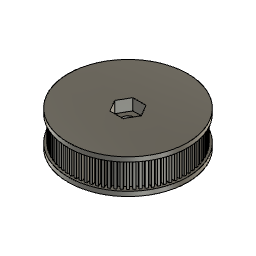
pulley5080 (Autodesk Fusion 360 design; units mm, degrees)
Autodesk Fusion 360 part; units mm, degrees
sketch "Sketch1" plane through (0, 0, 0) normal (0, 0, 1) x (1, 0, 0)
  line L0 (0.5, 23.5) -> (0.5, 25)
  line L1 (0.5, 25) -> (-0.5, 25)
  line L2 (-0.5, 25) -> (-0.5, 23.5)
  line L3 (0, 1.75) -> (0, 22.5)
  circle A0 centre (0, 0) radius 23.5053
  line L4 (-2.4599, 24.8837) -> (-2.3422, 23.3883)
  line L5 (-1.463, 24.9622) -> (-2.4599, 24.8837)
  line L6 (-1.3453, 23.4668) -> (-1.463, 24.9622)
  line L7 (-4.4047, 24.614) -> (-4.1701, 23.1325)
  line L8 (-3.417, 24.7704) -> (-4.4047, 24.614)
  line L9 (-3.1824, 23.2889) -> (-3.417, 24.7704)
  line L10 (-6.3223, 24.1925) -> (-5.9722, 22.734)
  line L11 (-5.3499, 24.426) -> (-6.3223, 24.1925)
  line L12 (-4.9998, 22.9674) -> (-5.3499, 24.426)
  line L13 (-8.201, 23.6219) -> (-7.7374, 22.1953)
  line L14 (-7.2499, 23.9309) -> (-8.201, 23.6219)
  line L15 (-6.7864, 22.5043) -> (-7.2499, 23.9309)
  line L16 (-10.029, 22.9056) -> (-9.455, 21.5198)
  line L17 (-9.1051, 23.2883) -> (-10.029, 22.9056)
  line L18 (-8.5311, 21.9025) -> (-9.1051, 23.2883)
  line L19 (-11.7953, 22.0482) -> (-11.1143, 20.7117)
  line L20 (-10.9043, 22.5022) -> (-11.7953, 22.0482)
  line L21 (-10.2233, 21.1656) -> (-10.9043, 22.5022)
  line L22 (-13.4888, 21.0548) -> (-12.705, 19.7758)
  line L23 (-12.6361, 21.5773) -> (-13.4888, 21.0548)
  line L24 (-11.8524, 20.2983) -> (-12.6361, 21.5773)
  line L25 (-15.0991, 19.9315) -> (-14.2175, 18.718)
  line L26 (-14.2901, 20.5193) -> (-15.0991, 19.9315)
  line L27 (-13.4084, 19.3058) -> (-14.2901, 20.5193)
  line L28 (-16.6164, 18.6854) -> (-15.6422, 17.5448)
  line L29 (-15.856, 19.3349) -> (-16.6164, 18.6854)
  line L30 (-14.8818, 18.1943) -> (-15.856, 19.3349)
  line L31 (-18.0312, 17.3241) -> (-16.9706, 16.2635)
  line L32 (-17.3241, 18.0312) -> (-18.0312, 17.3241)
  line L33 (-16.2635, 16.9706) -> (-17.3241, 18.0312)
  line L34 (-19.3349, 15.856) -> (-18.1943, 14.8818)
  line L35 (-18.6854, 16.6164) -> (-19.3349, 15.856)
  line L36 (-17.5448, 15.6422) -> (-18.6854, 16.6164)
  line L37 (-20.5193, 14.2901) -> (-19.3058, 13.4084)
  line L38 (-19.9315, 15.0991) -> (-20.5193, 14.2901)
  line L39 (-18.718, 14.2175) -> (-19.9315, 15.0991)
  line L40 (-21.5773, 12.6361) -> (-20.2983, 11.8524)
  line L41 (-21.0548, 13.4888) -> (-21.5773, 12.6361)
  line L42 (-19.7758, 12.705) -> (-21.0548, 13.4888)
  line L43 (-22.5022, 10.9043) -> (-21.1656, 10.2233)
  line L44 (-22.0482, 11.7953) -> (-22.5022, 10.9043)
  line L45 (-20.7117, 11.1143) -> (-22.0482, 11.7953)
  line L46 (-23.2883, 9.1051) -> (-21.9025, 8.5311)
  line L47 (-22.9056, 10.029) -> (-23.2883, 9.1051)
  line L48 (-21.5198, 9.455) -> (-22.9056, 10.029)
  line L49 (-23.9309, 7.2499) -> (-22.5043, 6.7864)
  line L50 (-23.6219, 8.201) -> (-23.9309, 7.2499)
  line L51 (-22.1953, 7.7374) -> (-23.6219, 8.201)
  line L52 (-24.426, 5.3499) -> (-22.9674, 4.9998)
  line L53 (-24.1925, 6.3223) -> (-24.426, 5.3499)
  line L54 (-22.734, 5.9722) -> (-24.1925, 6.3223)
  line L55 (-24.7704, 3.417) -> (-23.2889, 3.1824)
  line L56 (-24.614, 4.4047) -> (-24.7704, 3.417)
  line L57 (-23.1325, 4.1701) -> (-24.614, 4.4047)
  line L58 (-24.9622, 1.463) -> (-23.4668, 1.3453)
  line L59 (-24.8837, 2.4599) -> (-24.9622, 1.463)
  line L60 (-23.3883, 2.3422) -> (-24.8837, 2.4599)
  line L61 (-25, -0.5) -> (-23.5, -0.5)
  line L62 (-25, 0.5) -> (-25, -0.5)
  line L63 (-23.5, 0.5) -> (-25, 0.5)
  line L64 (-24.8837, -2.4599) -> (-23.3883, -2.3422)
  line L65 (-24.9622, -1.463) -> (-24.8837, -2.4599)
  line L66 (-23.4668, -1.3453) -> (-24.9622, -1.463)
  line L67 (-24.614, -4.4047) -> (-23.1325, -4.1701)
  line L68 (-24.7704, -3.417) -> (-24.614, -4.4047)
  line L69 (-23.2889, -3.1824) -> (-24.7704, -3.417)
  line L70 (-24.1925, -6.3223) -> (-22.734, -5.9722)
  line L71 (-24.426, -5.3499) -> (-24.1925, -6.3223)
  line L72 (-22.9674, -4.9998) -> (-24.426, -5.3499)
  line L73 (-23.6219, -8.201) -> (-22.1953, -7.7374)
  line L74 (-23.9309, -7.2499) -> (-23.6219, -8.201)
  line L75 (-22.5043, -6.7864) -> (-23.9309, -7.2499)
  line L76 (-22.9056, -10.029) -> (-21.5198, -9.455)
  line L77 (-23.2883, -9.1051) -> (-22.9056, -10.029)
  line L78 (-21.9025, -8.5311) -> (-23.2883, -9.1051)
  line L79 (-22.0482, -11.7953) -> (-20.7117, -11.1143)
  line L80 (-22.5022, -10.9043) -> (-22.0482, -11.7953)
  line L81 (-21.1656, -10.2233) -> (-22.5022, -10.9043)
  line L82 (-21.0548, -13.4888) -> (-19.7758, -12.705)
  line L83 (-21.5773, -12.6361) -> (-21.0548, -13.4888)
  line L84 (-20.2983, -11.8524) -> (-21.5773, -12.6361)
  line L85 (-19.9315, -15.0991) -> (-18.718, -14.2175)
  line L86 (-20.5193, -14.2901) -> (-19.9315, -15.0991)
  line L87 (-19.3058, -13.4084) -> (-20.5193, -14.2901)
  line L88 (-18.6854, -16.6164) -> (-17.5448, -15.6422)
  line L89 (-19.3349, -15.856) -> (-18.6854, -16.6164)
  line L90 (-18.1943, -14.8818) -> (-19.3349, -15.856)
  line L91 (-17.3241, -18.0312) -> (-16.2635, -16.9706)
  line L92 (-18.0312, -17.3241) -> (-17.3241, -18.0312)
  line L93 (-16.9706, -16.2635) -> (-18.0312, -17.3241)
  line L94 (-15.856, -19.3349) -> (-14.8818, -18.1943)
  line L95 (-16.6164, -18.6854) -> (-15.856, -19.3349)
  line L96 (-15.6422, -17.5448) -> (-16.6164, -18.6854)
  line L97 (-14.2901, -20.5193) -> (-13.4084, -19.3058)
  line L98 (-15.0991, -19.9315) -> (-14.2901, -20.5193)
  line L99 (-14.2175, -18.718) -> (-15.0991, -19.9315)
  line L100 (-12.6361, -21.5773) -> (-11.8524, -20.2983)
  line L101 (-13.4888, -21.0548) -> (-12.6361, -21.5773)
  line L102 (-12.705, -19.7758) -> (-13.4888, -21.0548)
  line L103 (-10.9043, -22.5022) -> (-10.2233, -21.1656)
  line L104 (-11.7953, -22.0482) -> (-10.9043, -22.5022)
  line L105 (-11.1143, -20.7117) -> (-11.7953, -22.0482)
  line L106 (-9.1051, -23.2883) -> (-8.5311, -21.9025)
  line L107 (-10.029, -22.9056) -> (-9.1051, -23.2883)
  line L108 (-9.455, -21.5198) -> (-10.029, -22.9056)
  line L109 (-7.2499, -23.9309) -> (-6.7864, -22.5043)
  line L110 (-8.201, -23.6219) -> (-7.2499, -23.9309)
  line L111 (-7.7374, -22.1953) -> (-8.201, -23.6219)
  line L112 (-5.3499, -24.426) -> (-4.9998, -22.9674)
  line L113 (-6.3223, -24.1925) -> (-5.3499, -24.426)
  line L114 (-5.9722, -22.734) -> (-6.3223, -24.1925)
  line L115 (-3.417, -24.7704) -> (-3.1824, -23.2889)
  line L116 (-4.4047, -24.614) -> (-3.417, -24.7704)
  line L117 (-4.1701, -23.1325) -> (-4.4047, -24.614)
  line L118 (-1.463, -24.9622) -> (-1.3453, -23.4668)
  line L119 (-2.4599, -24.8837) -> (-1.463, -24.9622)
  line L120 (-2.3422, -23.3883) -> (-2.4599, -24.8837)
  line L121 (0.5, -25) -> (0.5, -23.5)
  line L122 (-0.5, -25) -> (0.5, -25)
  line L123 (-0.5, -23.5) -> (-0.5, -25)
  line L124 (2.4599, -24.8837) -> (2.3422, -23.3883)
  line L125 (1.463, -24.9622) -> (2.4599, -24.8837)
  line L126 (1.3453, -23.4668) -> (1.463, -24.9622)
  line L127 (4.4047, -24.614) -> (4.1701, -23.1325)
  line L128 (3.417, -24.7704) -> (4.4047, -24.614)
  line L129 (3.1824, -23.2889) -> (3.417, -24.7704)
  line L130 (6.3223, -24.1925) -> (5.9722, -22.734)
  line L131 (5.3499, -24.426) -> (6.3223, -24.1925)
  line L132 (4.9998, -22.9674) -> (5.3499, -24.426)
  line L133 (8.201, -23.6219) -> (7.7374, -22.1953)
  line L134 (7.2499, -23.9309) -> (8.201, -23.6219)
  line L135 (6.7864, -22.5043) -> (7.2499, -23.9309)
  line L136 (10.029, -22.9056) -> (9.455, -21.5198)
  line L137 (9.1051, -23.2883) -> (10.029, -22.9056)
  line L138 (8.5311, -21.9025) -> (9.1051, -23.2883)
  line L139 (11.7953, -22.0482) -> (11.1143, -20.7117)
  line L140 (10.9043, -22.5022) -> (11.7953, -22.0482)
  line L141 (10.2233, -21.1656) -> (10.9043, -22.5022)
  line L142 (13.4888, -21.0548) -> (12.705, -19.7758)
  line L143 (12.6361, -21.5773) -> (13.4888, -21.0548)
  line L144 (11.8524, -20.2983) -> (12.6361, -21.5773)
  line L145 (15.0991, -19.9315) -> (14.2175, -18.718)
  line L146 (14.2901, -20.5193) -> (15.0991, -19.9315)
  line L147 (13.4084, -19.3058) -> (14.2901, -20.5193)
  line L148 (16.6164, -18.6854) -> (15.6422, -17.5448)
  line L149 (15.856, -19.3349) -> (16.6164, -18.6854)
  line L150 (14.8818, -18.1943) -> (15.856, -19.3349)
  line L151 (18.0312, -17.3241) -> (16.9706, -16.2635)
  line L152 (17.3241, -18.0312) -> (18.0312, -17.3241)
  line L153 (16.2635, -16.9706) -> (17.3241, -18.0312)
  line L154 (19.3349, -15.856) -> (18.1943, -14.8818)
  line L155 (18.6854, -16.6164) -> (19.3349, -15.856)
  line L156 (17.5448, -15.6422) -> (18.6854, -16.6164)
  line L157 (20.5193, -14.2901) -> (19.3058, -13.4084)
  line L158 (19.9315, -15.0991) -> (20.5193, -14.2901)
  line L159 (18.718, -14.2175) -> (19.9315, -15.0991)
  line L160 (21.5773, -12.6361) -> (20.2983, -11.8524)
  line L161 (21.0548, -13.4888) -> (21.5773, -12.6361)
  line L162 (19.7758, -12.705) -> (21.0548, -13.4888)
  line L163 (22.5022, -10.9043) -> (21.1656, -10.2233)
  line L164 (22.0482, -11.7953) -> (22.5022, -10.9043)
  line L165 (20.7117, -11.1143) -> (22.0482, -11.7953)
  line L166 (23.2883, -9.1051) -> (21.9025, -8.5311)
  line L167 (22.9056, -10.029) -> (23.2883, -9.1051)
  line L168 (21.5198, -9.455) -> (22.9056, -10.029)
  line L169 (23.9309, -7.2499) -> (22.5043, -6.7864)
  line L170 (23.6219, -8.201) -> (23.9309, -7.2499)
  line L171 (22.1953, -7.7374) -> (23.6219, -8.201)
  line L172 (24.426, -5.3499) -> (22.9674, -4.9998)
  line L173 (24.1925, -6.3223) -> (24.426, -5.3499)
  line L174 (22.734, -5.9722) -> (24.1925, -6.3223)
  line L175 (24.7704, -3.417) -> (23.2889, -3.1824)
  line L176 (24.614, -4.4047) -> (24.7704, -3.417)
  line L177 (23.1325, -4.1701) -> (24.614, -4.4047)
  line L178 (24.9622, -1.463) -> (23.4668, -1.3453)
  line L179 (24.8837, -2.4599) -> (24.9622, -1.463)
  line L180 (23.3883, -2.3422) -> (24.8837, -2.4599)
  line L181 (25, 0.5) -> (23.5, 0.5)
  line L182 (25, -0.5) -> (25, 0.5)
  line L183 (23.5, -0.5) -> (25, -0.5)
  line L184 (24.8837, 2.4599) -> (23.3883, 2.3422)
  line L185 (24.9622, 1.463) -> (24.8837, 2.4599)
  line L186 (23.4668, 1.3453) -> (24.9622, 1.463)
  line L187 (24.614, 4.4047) -> (23.1325, 4.1701)
  line L188 (24.7704, 3.417) -> (24.614, 4.4047)
  line L189 (23.2889, 3.1824) -> (24.7704, 3.417)
  line L190 (24.1925, 6.3223) -> (22.734, 5.9722)
  line L191 (24.426, 5.3499) -> (24.1925, 6.3223)
  line L192 (22.9674, 4.9998) -> (24.426, 5.3499)
  line L193 (23.6219, 8.201) -> (22.1953, 7.7374)
  line L194 (23.9309, 7.2499) -> (23.6219, 8.201)
  line L195 (22.5043, 6.7864) -> (23.9309, 7.2499)
  line L196 (22.9056, 10.029) -> (21.5198, 9.455)
  line L197 (23.2883, 9.1051) -> (22.9056, 10.029)
  line L198 (21.9025, 8.5311) -> (23.2883, 9.1051)
  line L199 (22.0482, 11.7953) -> (20.7117, 11.1143)
  line L200 (22.5022, 10.9043) -> (22.0482, 11.7953)
  line L201 (21.1656, 10.2233) -> (22.5022, 10.9043)
  line L202 (21.0548, 13.4888) -> (19.7758, 12.705)
  line L203 (21.5773, 12.6361) -> (21.0548, 13.4888)
  line L204 (20.2983, 11.8524) -> (21.5773, 12.6361)
  line L205 (19.9315, 15.0991) -> (18.718, 14.2175)
  line L206 (20.5193, 14.2901) -> (19.9315, 15.0991)
  line L207 (19.3058, 13.4084) -> (20.5193, 14.2901)
  line L208 (18.6854, 16.6164) -> (17.5448, 15.6422)
  line L209 (19.3349, 15.856) -> (18.6854, 16.6164)
  line L210 (18.1943, 14.8818) -> (19.3349, 15.856)
  line L211 (17.3241, 18.0312) -> (16.2635, 16.9706)
  line L212 (18.0312, 17.3241) -> (17.3241, 18.0312)
  line L213 (16.9706, 16.2635) -> (18.0312, 17.3241)
  line L214 (15.856, 19.3349) -> (14.8818, 18.1943)
  line L215 (16.6164, 18.6854) -> (15.856, 19.3349)
  line L216 (15.6422, 17.5448) -> (16.6164, 18.6854)
  line L217 (14.2901, 20.5193) -> (13.4084, 19.3058)
  line L218 (15.0991, 19.9315) -> (14.2901, 20.5193)
  line L219 (14.2175, 18.718) -> (15.0991, 19.9315)
  line L220 (12.6361, 21.5773) -> (11.8524, 20.2983)
  line L221 (13.4888, 21.0548) -> (12.6361, 21.5773)
  line L222 (12.705, 19.7758) -> (13.4888, 21.0548)
  line L223 (10.9043, 22.5022) -> (10.2233, 21.1656)
  line L224 (11.7953, 22.0482) -> (10.9043, 22.5022)
  line L225 (11.1143, 20.7117) -> (11.7953, 22.0482)
  line L226 (9.1051, 23.2883) -> (8.5311, 21.9025)
  line L227 (10.029, 22.9056) -> (9.1051, 23.2883)
  line L228 (9.455, 21.5198) -> (10.029, 22.9056)
  line L229 (7.2499, 23.9309) -> (6.7864, 22.5043)
  line L230 (8.201, 23.6219) -> (7.2499, 23.9309)
  line L231 (7.7374, 22.1953) -> (8.201, 23.6219)
  line L232 (5.3499, 24.426) -> (4.9998, 22.9674)
  line L233 (6.3223, 24.1925) -> (5.3499, 24.426)
  line L234 (5.9722, 22.734) -> (6.3223, 24.1925)
  line L235 (3.417, 24.7704) -> (3.1824, 23.2889)
  line L236 (4.4047, 24.614) -> (3.417, 24.7704)
  line L237 (4.1701, 23.1325) -> (4.4047, 24.614)
  line L238 (1.463, 24.9622) -> (1.3453, 23.4668)
  line L239 (2.4599, 24.8837) -> (1.463, 24.9622)
  line L240 (2.3422, 23.3883) -> (2.4599, 24.8837)
  circle A1 centre (0, 0) radius 26
  dimension "d1" = 1
  dimension "d2" = 1.5
  dimension "d3" = 25
  dimension "d5" = 360
  dimension "d6" = 52
  constraint vertical L0
  constraint horizontal L1
  constraint vertical L2
  constraint symmetric L2.end L0.start L3
  constraint coincident A0.centre A1.centre
  constraint coincident L2.end A0
  measures "d1" distance of L0.end L1.end
  measures "d2" distance of L0.start L0.end
  measures "d3" distance of A0.centre L1
  measures "d6" diameter of A1
extrude "Extrude1" add sketch "Sketch1" along normal blind 15 contours L0 L1 L2 A0 | A0 | A0 L238 L239 L240 | A0 L4 L5 L6 | A0 L235 L236 L237 | A0 L7 L8 L9 | A0 L232 L233 L234 | A0 L10 L11 L12 | A0 L229 L230 L231 | A0 L13 L14 L15 | A0 L226 L227 L228 | A0 L16 L17 L18 | A0 L223 L224 L225 | A0 L19 L20 L21 | A0 L220 L221 L222 | A0 L22 L23 L24 | A0 L217 L218 L219 | A0 L25 L26 L27 | A0 L214 L215 L216 | A0 L28 L29 L30 | A0 L211 L212 L213 | A0 L31 L32 L33 | A0 L208 L209 L210 | A0 L34 L35 L36 | A0 L205 L206 L207 | A0 L37 L38 L39 | A0 L202 L203 L204 | A0 L40 L41 L42 | A0 L199 L200 L201 | A0 L43 L44 L45 | A0 L196 L197 L198 | A0 L46 L47 L48 | A0 L193 L194 L195 | A0 L49 L50 L51 | A0 L190 L191 L192 | A0 L52 L53 L54 | A0 L187 L188 L189 | A0 L55 L56 L57 | A0 L184 L185 L186 | A0 L58 L59 L60 | A0 L181 L182 L183 | A0 L61 L62 L63 | A0 L178 L179 L180 | A0 L64 L65 L66 | A0 L175 L176 L177 | A0 L67 L68 L69 | A0 L172 L173 L174 | A0 L70 L71 L72 | A0 L169 L170 L171 | A0 L73 L74 L75 | A0 L166 L167 L168 | A0 L76 L77 L78 | A0 L163 L164 L165 | A0 L79 L80 L81 | A0 L160 L161 L162 | A0 L82 L83 L84 | A0 L157 L158 L159 | A0 L85 L86 L87 | A0 L154 L155 L156 | A0 L88 L89 L90 | A0 L151 L152 L153 | A0 L91 L92 L93 | A0 L148 L149 L150 | A0 L94 L95 L96 | A0 L145 L146 L147 | A0 L97 L98 L99 | A0 L142 L143 L144 | A0 L100 L101 L102 | A0 L139 L140 L141 | A0 L103 L104 L105 | A0 L136 L137 L138 | A0 L106 L107 L108 | A0 L133 L134 L135 | A0 L109 L110 L111 | A0 L130 L131 L132 | A0 L112 L113 L114 | A0 L127 L128 L129 | A0 L115 L116 L117 | A0 L124 L125 L126 | A0 L118 L119 L120 | A0 L121 L122 L123
extrude "Extrude2" add sketch "Sketch1" along normal blind 2
extrude "Extrude3" add sketch "Sketch1" against normal blind 2 from surface at 15
sketch "Sketch2" plane through (0, 0, 15) normal (0, 0, 1) x (-1, 0, 0)
  circle A0 centre (0, 0) radius 26
  circle A1 centre (0, 0) radius 3
  line L0 (2.8868, -5) -> (5.7735, 0)
  line L1 (5.7735, 0) -> (2.8868, 5)
  line L2 (2.8868, 5) -> (-2.8868, 5)
  line L3 (-2.8868, 5) -> (-5.7735, 0)
  line L4 (-5.7735, 0) -> (-2.8868, -5)
  line L5 (-2.8868, -5) -> (2.8868, -5)
  dimension "d14" = 6
  dimension "d15" = 10
  constraint coincident A0.centre A1.centre
  constraint horizontal L5
  measures "d14" diameter of A1
  measures "d15" distance of L2 L5
extrude "Extrude4" cut sketch "Sketch2" against normal through all contours A1
extrude "Extrude5" cut sketch "Sketch2" against normal blind 5 contours L0 L1 L2 L3 L4 L5
